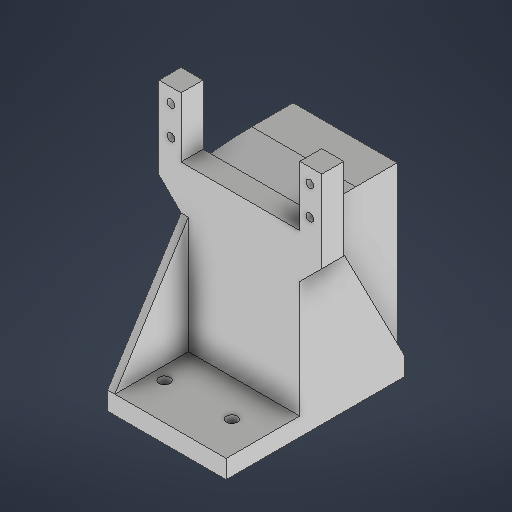
# Autodesk Inventor part: ServoMountV1
Saved by Autodesk Inventor 2025.1 (Build 291241020, 241B)
## iProperties
Created: 2025-04-20
Part Number: ServoMountV1
Material: Generic
Document SubType Name: Modeling
Designer: dpseu
Density: 1 g/cm^3
Appearance: Default
Author: dpseu
Autodesk Inventor part; units mm, degrees
ref_plane "YZ Plane" through (0, 0, 0) normal (1, 0, 0) x (0, 1, 0)
ref_plane "XZ Plane" through (0, 0, 0) normal (0, 1, 0) x (-1, 0, 0)
ref_plane "XY Plane" through (0, 0, 0) normal (0, 0, 1) x (1, 0, 0)
sketch "Sketch1" plane through (0, 0, 0) normal (0, 0, 1) x (1, 0, 0)
  line L0 (56.261, 7.62) -> (56.261, 35.941)
  line L1 (56.261, 35.941) -> (0, 35.941)
  line L2 (0, 35.941) -> (0, 7.62)
  line L3 (7.62, 28.321) -> (48.641, 28.321)
  line L4 (48.641, 28.321) -> (48.641, 7.62)
  line L5 (7.62, 7.62) -> (7.62, 28.321)
  line L6 (7.62, 7.62) -> (0, 7.62)
  line L7 (48.641, 7.62) -> (56.261, 7.62)
  circle A0 centre (52.141, 12.62) radius 1.3525
  circle A1 centre (52.141, 22.62) radius 1.3525
  circle A2 centre (4.12, 22.62) radius 1.3525
  circle A3 centre (4.12, 12.62) radius 1.3525
  line L8 (7.62, 35.941) -> (48.641, 35.941)
  line L9 (48.641, 35.941) -> (48.641, 90.1751)
  line L10 (48.641, 90.1751) -> (7.62, 90.1751)
  line L11 (7.62, 90.1751) -> (7.62, 35.941)
  line L12 (0, 35.941) -> (7.62, 43.561)
  line L13 (0, 35.941) -> (10.7763, 35.941) construction
  line L14 (56.261, 35.941) -> (48.641, 43.561)
  line L15 (56.261, 35.941) -> (67.0373, 35.941) construction
  point P0 (0, 0)
  dimension "d24" = 56.261
  dimension "d28" = 7.62
  dimension "d29" = 7.62
  dimension "d30" = 28.321
  dimension "d31" = 7.62
  dimension "d32" = 2.7051
  dimension "d33" = 3.5
  dimension "d34" = 2.7051
  dimension "d35" = 3.5
  dimension "d36" = 5
  dimension "d37" = 15
  dimension "d38" = 2.7051
  dimension "d39" = 2.7051
  dimension "d40" = 3.5
  dimension "d41" = 3.5
  dimension "d42" = 15
  dimension "d43" = 5
  dimension "d44" = 41.021
  dimension "d52" = 54.2341
  dimension "d53" = 45
  dimension "d54" = 135
  constraints: 32 end point, 4 centre point, 4 horizontal, 4 parallel, 4 point on line, 3 perpendicular, 2 equal length
  measures "d24" distance of L1.end L0.end
  measures "d28" distance between parallel lines of L2 L5
  measures "d29" distance between parallel lines of L1 L3
  measures "d30" distance of L0.start L0.end
  measures "d31" distance of L4.end L0.start
  measures "d32" diameter of A0
  measures "d33" distance from line of L4 A0.centre
  measures "d34" diameter of A1
  measures "d35" distance from line of L4 A1.centre
  measures "d36" distance from line of L7 A0.centre
  measures "d37" distance from line of L7 A1.centre
  measures "d38" diameter of A3
  measures "d39" diameter of A2
  measures "d40" distance from line of L5 A3.centre
  measures "d41" distance from line of L5 A2.centre
  measures "d42" distance from line of A2.centre L6
  measures "d43" distance from line of L6 A3.centre
  measures "d44" distance of L10.end L9.end
  measures "d52" distance of L8.end L9.end
  measures "d53" angle of L13 L12
  measures "d54" angle of L15 L14
extrude "Extrusion1" add sketch "Sketch1" along normal blind 7.62
sketch "Sketch2" plane through (7.62, 90.1751, 0) normal (0, 1, 0) x (1, 0, 0)
  line L0 (41.021, -7.62) -> (0, -7.62) projected
  line L1 (0, -7.62) -> (41.021, -7.62)
  line L2 (41.021, -7.62) -> (41.021, 25.4)
  line L3 (41.021, 25.4) -> (0, 25.4)
  line L4 (0, 25.4) -> (0, -7.62)
  circle A0 centre (6.985, 12.7) radius 1.905
  circle A1 centre (30.226, 12.7) radius 1.905
  line L5 (0, 0) -> (-7.62, 0) projected
  line L6 (41.021, 0) -> (0, 0) projected
  line L7 (0, 0) -> (41.021, 0)
  point P0 (-7.62, -7.62)
  dimension "d65" = 33.02
  dimension "d66" = 41.021
  dimension "d67" = 3.81
  dimension "d68" = 3.81
  dimension "d69" = 12.7
  dimension "d70" = 12.7
  dimension "d71" = 6.985
  dimension "d72" = 10.795
  constraints: 10 end point, 3 equal length, 2 centre point, 1 horizontal, 1 perpendicular
  measures "d65" distance of L2.end L1.end
  measures "d66" distance of L2.end L3.end
  measures "d67" diameter of A0
  measures "d68" diameter of A1
  measures "d69" distance from line of L3 A0.centre
  measures "d70" distance from line of L3 A1.centre
  measures "d71" distance from line of L4 A0.centre
  measures "d72" distance from line of L2 A1.centre
extrude "Extrusion2" add sketch "Sketch2" against normal blind 6.35 contours L6 L4 L3 L2
sketch "Sketch3" plane through (7.62, 43.561, 7.62) normal (-1, 0, 0) x (0, 0, 1)
  line L0 (-7.62, 0) -> (0, 0) projected
  line L1 (-33.02, 40.2641) -> (-7.62, 40.2641) projected
  line L2 (-7.62, 0) -> (-33.02, 40.2641)
  line L3 (-33.02, 40.2641) -> (-7.62, 40.2641)
  line L4 (-7.62, 40.2641) -> (-7.62, 0)
  point P0 (-7.62, -43.561)
  constraints: 6 end point, 1 collinear, 1 perpendicular
extrude "Extrusion3" add sketch "Sketch3" against normal blind 2.54
sketch "Sketch4" plane through (48.641, 43.561, 7.62) normal (1, 0, 0) x (0, 0, -1)
  line L0 (7.62, -35.941) -> (0, -35.941) projected
  line L1 (0, 46.6141) -> (-28.575, 46.6141)
  line L2 (-28.575, 46.6141) -> (-28.575, 40.2641)
  line L3 (0.6512, -16.5049) -> (0, -16.5049)
  line L4 (0, -16.5049) -> (0, 46.6141)
  line L5 (0, 40.2641) -> (-28.575, 40.2641)
  line L6 (7.62, -15.24) -> (0, -15.24) projected
  line L7 (0, -15.24) -> (-28.575, 40.2641)
  point P0 (7.62, -43.561)
  dimension "d99" = 6.35
  dimension "d102" = 28.575
  dimension "d103" = 63.119
  constraints: 12 end point, 2 parallel, 2 perpendicular, 2 point on line, 1 horizontal
  measures "d99" distance between parallel lines of L1 L5
  measures "d102" distance of L1.start L1.end
  measures "d103" distance of L3.end L1.start
extrude "Extrusion6" add sketch "Sketch4" against normal blind 2.54
extrude "Extrusion7" add sketch "Sketch4" against normal blind 41.021 contours L4 L5 L2 L1
sketch "Sketch7" plane through (7.62, 83.8251, -25.4) normal (-1, 0, 0) x (0, 0, 1)
  line L0 (33.02, 0) -> (61.595, 0)
  line L1 (33.02, -55.499) -> (33.02, 0)
  line L2 (61.595, 0) -> (33.02, -55.499)
  point P0 (25.4, -83.8251)
  dimension "d111" = 55.499
  dimension "d112" = 28.575
  dimension "d113" = 90
  constraints: 6 end point, 1 horizontal
  measures "d111" distance of L1.start L0.start
  measures "d112" distance of L0.start L0.end
  measures "d113" angle of L0 L1
extrude "Extrusion8" add sketch "Sketch7" against normal blind 2.54
sketch "Sketch10" plane through (46.101, 83.8251, 7.62) normal (0, -1, 0) x (1, 0, 0)
  line L0 (-35.941, 28.575) -> (-35.941, 0) projected
  line L1 (0, 0) -> (-35.941, 0)
  line L2 (-35.941, 0) -> (-35.941, 28.575)
  line L3 (-35.941, 28.575) -> (0, 28.575)
  line L4 (0, 28.575) -> (0, 0)
  point P0 (-46.101, -7.62)
  point P1 (-35.941, 0)
  constraints: 8 end point, 2 parallel, 1 horizontal, 1 perpendicular
extrude "Extrusion11" add sketch "Sketch10" along normal blind 56.388
fillet "Fillet1" radius 115.57 1 edges at (28.1305, 27.4371, 7.62)
body "Solid1"
